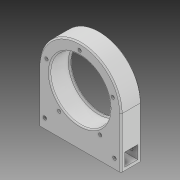
# Autodesk Inventor part: TestBracket
Saved by Autodesk Inventor 2020 (Build 240168000, 168)
## iProperties
Created: 2021-03-20
Part Number: TestBracket
Material: Generic
Document SubType Name: Modeling
Designer: DDeGo
Density: 1 g/cm^3
Appearance: Default
Author: DDeGo
Autodesk Inventor part; units mm, degrees
ref_plane "YZ Plane" through (0, 0, 0) normal (1, 0, 0) x (0, 1, 0)
ref_plane "XZ Plane" through (0, 0, 0) normal (0, 1, 0) x (-1, 0, 0)
sketch "Sketch1" plane through (0, 0, 0) normal (0, 0, 1) x (1, 0, 0)
  circle A0 centre (0, 0) radius 47.525
  arc A1 (65, 0) -> (-65, 0) centre (0, 0) ccw
  line L0 (-65, 0) -> (-65, -80)
  line L1 (-65, -80) -> (65, -80)
  line L2 (65, -80) -> (65, 0)
  dimension "d0" = 95.05
  dimension "d2" = 80
  dimension "d43" = 65
  constraints: 6 end point, 2 centre point, 2 coincident, 2 point on circle, 2 tangent, 2 vertical, 1 perpendicular
  measures "d0" diameter of A0
  measures "d2" distance from line of L1 point (0, 0)
  measures "d43" radius of A1
extrude "Extrusion1" add sketch "Sketch1" along normal blind 32.5
sketch "Sketch2" plane through (0, 0, 0) normal (0, 0, -1) x (-1, 0, 0)
  circle A0 centre (0, 0) radius 47.525 projected
  circle A1 centre (0, 0) radius 45.525
  dimension "d5" = 2
  constraints: 1 centre point, 1 coincident
  measures "d5" radial gap between concentric circles of A0 A1
extrude "Extrusion2" add sketch "Sketch2" against normal blind 1
sketch "Sketch3" plane through (0, 0, 32.5) normal (0, 0, 1) x (1, 0, 0)
  arc A0 (65, 0) -> (-65, 0) centre (0, 0) ccw construction
  line L0 (0, 0) -> (0, 55) construction
  circle A1 centre (0, 55) radius 2.6
  circle A2 centre (-52.3081, 16.9959) radius 2.6
  circle A3 centre (-32.3282, -44.4959) radius 2.6
  circle A4 centre (32.3282, -44.4959) radius 2.6
  circle A5 centre (52.3081, 16.9959) radius 2.6
  dimension "d8" = 5.2
  dimension "d9" = 55
  dimension "d12" = 360
  constraints: 5 centre point, 5 coincident, 2 end point, 1 vertical, 16 other
  measures "d8" diameter of A1
  measures "d9" distance of L0.start L0.end
extrude "Extrusion3" cut sketch "Sketch3" against normal through all
ref_plane "Work Plane1" through (-65, -65, 0) normal (0, -1, 0) x (1, 0, 0)
fillet "Fillet1" radius 2 1 edges at (-47.525, 0, 32.5)
chamfer "Chamfer1" distance 2 angle 45 6 edges at (0, 65, 32.5) (-65, -40, 32.5) (65, -40, 32.5) (0, 65, 0) (-65, -40, 0) (65, -40, 0)
chamfer "Chamfer2" distance 2 angle 45 1 edges at (-47.525, 0, 1)
sketch "Sketch9" plane through (65, -80, 2) normal (1, 0, 0) x (0, 0, -1)
  line L0 (0, 0) -> (-28.5, 0) construction
  line L1 (-14.25, 0) -> (-14.25, 15) construction
  line L2 (-24.5, 25.25) -> (-4, 25.25)
  line L3 (-4, 25.25) -> (-4, 4.75)
  line L4 (-4, 4.75) -> (-24.5, 4.75)
  line L5 (-24.5, 4.75) -> (-24.5, 25.25)
  line L6 (-24.5, 25.25) -> (-4, 4.75) construction
  line L7 (-4, 25.25) -> (-24.5, 4.75) construction
  point P0 (2, 80)
  dimension "d48" = 20.5
  dimension "d49" = 20.5
  dimension "d50" = 15
  constraints: 14 end point, 3 midpoint, 2 parallel, 1 horizontal, 1 perpendicular, 1 vertical
  measures "d48" distance of L3.end L4.end
  measures "d49" distance of L2.end L3.end
  measures "d50" distance of L1.start L1.end
extrude "Extrusion8" cut sketch "Sketch9" against normal through all
sketch "Sketch10" plane through (0, 0, 0) normal (0, 0, -1) x (-1, 0, 0)
  line L0 (-65, -75.25) -> (-65, -54.75) projected
  line L1 (-65, -65) -> (65, -65) construction
  line L2 (65, -75.25) -> (65, -54.75) projected
  circle A0 centre (-55, -65) radius 2.75
  circle A1 centre (55, -65) radius 2.75
  point P0 (0, 0)
  dimension "d53" = 5.5
  dimension "d54" = 10
  dimension "d55" = 10
  constraints: 2 centre point, 2 end point, 2 midpoint, 2 point on line, 1 equal radius
  measures "d53" diameter of A0
  measures "d54" distance from line of A0.centre L0
  measures "d55" distance from line of L2 A1.centre
extrude "Extrusion9" cut sketch "Sketch10" against normal through all
sketch "Sketch11" plane through (0, 0, 0) normal (0, 0, -1) x (-1, 0, 0)
  circle A0 centre (0, 55) radius 2.6 construction
  line L0 (0, 50.208) -> (-4.15, 52.604)
  line L1 (-4.15, 52.604) -> (-4.15, 57.396)
  line L2 (-4.15, 57.396) -> (0, 59.792)
  line L3 (0, 59.792) -> (4.15, 57.396)
  line L4 (4.15, 57.396) -> (4.15, 52.604)
  line L5 (4.15, 52.604) -> (0, 50.208)
  line L6 (-47.7506, 15.5151) -> (-51.3118, 12.3086)
  line L7 (-51.3118, 12.3086) -> (-55.8693, 13.7895)
  line L8 (-55.8693, 13.7895) -> (-56.8656, 18.4767)
  line L9 (-56.8656, 18.4767) -> (-53.3044, 21.6832)
  line L10 (-53.3044, 21.6832) -> (-48.747, 20.2024)
  line L11 (-48.747, 20.2024) -> (-47.7506, 15.5151)
  line L12 (-29.5115, -40.6191) -> (-27.5624, -44.9968)
  line L13 (-27.5624, -44.9968) -> (-30.3791, -48.8737)
  line L14 (-30.3791, -48.8737) -> (-35.1449, -48.3727)
  line L15 (-35.1449, -48.3727) -> (-37.0939, -43.995)
  line L16 (-37.0939, -43.995) -> (-34.2773, -40.1182)
  line L17 (-34.2773, -40.1182) -> (-29.5115, -40.6191)
  line L18 (29.5115, -40.6191) -> (34.2773, -40.1182)
  line L19 (34.2773, -40.1182) -> (37.0939, -43.995)
  line L20 (37.0939, -43.995) -> (35.1449, -48.3727)
  line L21 (35.1449, -48.3727) -> (30.3791, -48.8737)
  line L22 (30.3791, -48.8737) -> (27.5624, -44.9968)
  line L23 (27.5624, -44.9968) -> (29.5115, -40.6191)
  line L24 (47.7506, 15.5151) -> (48.747, 20.2024)
  line L25 (48.747, 20.2024) -> (53.3044, 21.6832)
  line L26 (53.3044, 21.6832) -> (56.8656, 18.4767)
  line L27 (56.8656, 18.4767) -> (55.8693, 13.7895)
  line L28 (55.8693, 13.7895) -> (51.3118, 12.3086)
  line L29 (51.3118, 12.3086) -> (47.7506, 15.5151)
  point P0 (0, 0)
  point P1 (-52.3081, 16.9959)
  point P2 (-52.3081, 16.9959)
  point P3 (-32.3282, -44.4959)
  point P4 (-32.3282, -44.4959)
  point P5 (32.3282, -44.4959)
  point P6 (32.3282, -44.4959)
  point P7 (52.3081, 16.9959)
  point P8 (52.3081, 16.9959)
  dimension "d58" = 8.3
  dimension "d61" = 360
  constraints: 60 end point, 5 coincident, 1 vertical, 84 other
  measures "d58" distance between parallel lines of L4 L1
extrude "Extrusion10" cut sketch "Sketch11" against normal blind 15.25
body "Solid1"
